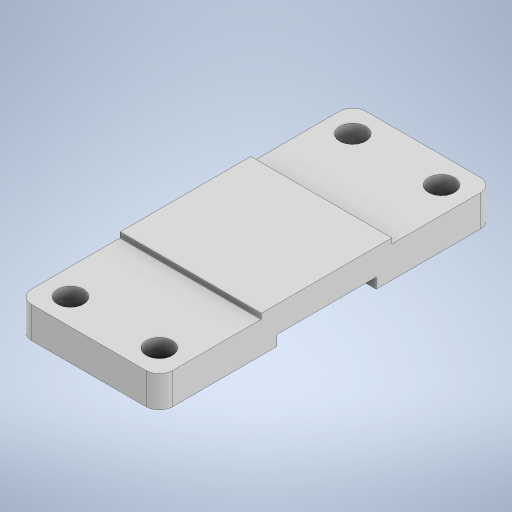
# Autodesk Inventor part: 4 - Part 5
Saved by Autodesk Inventor 2024 (Build 280153000, 153)
## iProperties
Created: 2024-04-20
Part Number: 4 - Part 5
Material: Generic
Document SubType Name: Modeling
Designer: Ricsi
Density: 1 g/cm^3
Appearance: Default
Author: Ricsi
Autodesk Inventor part; units mm, degrees
ref_plane "YZ Plane" through (0, 0, 0) normal (1, 0, 0) x (0, 1, 0)
ref_plane "XZ Plane" through (0, 0, 0) normal (0, 1, 0) x (-1, 0, 0)
ref_plane "XY Plane" through (0, 0, 0) normal (0, 0, 1) x (1, 0, 0)
sketch "Sketch1" plane through (0, 0, 0) normal (0, 1, 0) x (-1, 0, 0)
  line L0 (5, 0) -> (49, 0)
  line L1 (54, -5) -> (54, -123)
  line L2 (49, -128) -> (5, -128)
  line L3 (0, -123) -> (0, -5)
  arc A0 (5, 0) -> (0, -5) centre (5, -5) ccw
  arc A1 (54, -5) -> (49, 0) centre (49, -5) ccw
  arc A2 (49, -128) -> (54, -123) centre (49, -123) ccw
  arc A3 (0, -123) -> (5, -128) centre (5, -123) ccw
  circle A4 centre (44, -10) radius 5
  circle A5 centre (44, -118) radius 5
  circle A6 centre (10, -10) radius 5
  circle A7 centre (10, -118) radius 5
  point P0 (0, 0)
  point P1 (54, -128)
  point P2 (54, 0)
  point P3 (0, -128)
  dimension "d0" = 54
  dimension "d1" = 128
  dimension "d2" = 5
  dimension "d3" = 5
  dimension "d4" = 5
  dimension "d5" = 5
  dimension "d6" = 10
  dimension "d7" = 10
  dimension "d8" = 10
  dimension "d9" = 10
  dimension "d10" = 10
  dimension "d11" = 10
  dimension "d12" = 10
  dimension "d13" = 10
  dimension "d14" = 10
  dimension "d16" = 10
  dimension "d17" = 10
  dimension "d18" = 10
  constraints: 8 centre point, 8 end point, 8 point on circle, 8 point on line, 8 tangent, 2 parallel, 1 horizontal, 1 perpendicular
  measures "d0" distance of point (54, -128) point (0, -128)
  measures "d1" distance of point (54, 0) point (54, -128)
  measures "d2" radius of A0
  measures "d3" radius of A1
  measures "d4" radius of A2
  measures "d5" radius of A3
  measures "d6" diameter of A4
  measures "d7" distance from line of L0 A4.centre
  measures "d8" diameter of A5
  measures "d9" distance from line of A5.centre L2
  measures "d10" diameter of A6
  measures "d11" distance from line of L1 A4.centre
  measures "d12" distance from line of L3 A6.centre
  measures "d13" distance from line of L0 A6.centre
  measures "d14" distance from line of A5.centre L1
  measures "d16" diameter of A7
  measures "d17" distance from line of L2 A7.centre
  measures "d18" distance from line of L3 A7.centre
extrude "Extrusion1" add sketch "Sketch1" along normal blind 12
sketch "Sketch2" plane through (0, 0, -5) normal (1, 0, 0) x (0, 0, -1)
  line L0 (0, 0) -> (0, 12) projected
  line L1 (123, 0) -> (118, 0) projected
  line L2 (59, 0) -> (78, 0)
  line L3 (118, 0) -> (0, 0) projected
  line L4 (59, 0) -> (40, 0)
  line L5 (40, 0) -> (40, 4)
  line L6 (78, 0) -> (78, 4)
  line L7 (78, 4) -> (40, 4)
  point P0 (-5, 0)
  dimension "d22" = 19
  dimension "d23" = 19
  dimension "d24" = 4
  dimension "d25" = 4
  constraints: 10 end point, 2 perpendicular, 2 point on line, 1 vertical
  measures "d22" distance of L2.start L2.end
  measures "d23" distance of L2.start L4.end
  measures "d24" distance of L4.end L5.end
  measures "d25" distance of L2.end L6.end
extrude "Extrusion2" cut sketch "Sketch2" against normal blind 85.25
sketch "Sketch3" plane through (0, 12, 0) normal (0, 1, 0) x (1, 0, 0)
  line L0 (-54, 5) -> (-54, 64)
  line L1 (-54, 64) -> (-54, 89)
  line L2 (-54, 64) -> (-54, 39)
  line L3 (-54, 39) -> (0, 39)
  line L4 (0, 5) -> (0, 123) projected
  line L5 (-54, 89) -> (0, 89)
  line L6 (0, 39) -> (0, 89)
  point P0 (0, 0)
  dimension "d29" = 25
  dimension "d30" = 25
  constraints: 12 end point, 3 point on line, 1 collinear, 1 horizontal, 1 perpendicular
  measures "d29" distance of L0.end L1.end
  measures "d30" distance of L0.end L2.end
extrude "Extrusion3" add sketch "Sketch3" along normal blind 2
body "Solid1"
